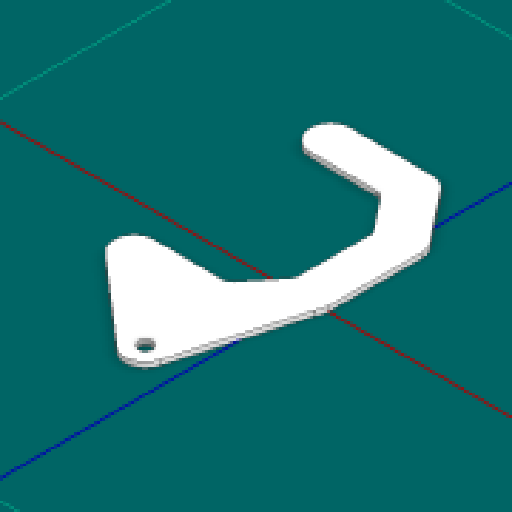
# Autodesk Inventor part: funnel_gusset
Saved by Autodesk Inventor 2025 (Build 290162000, 162)
## iProperties
Created: 2024-08-16
Part Number: funnel_gusset
Material: Acetal Resin, White
Document SubType Name: Modeling
Designer: averey
Density: 1.425 g/cm^3
Appearance: Smooth - White
d0: 0.500 in
d1: 0.500 in
d2: 0.500 in
d3: 0.125 in
d6: 0.176 in
d7: 0.176 in
d8: 0.176 in
d9: 0.176 in
d10: 0.500 in
d11: 0.500 in
d12: 0.250 in
d13: 0.250 in
d14: 0.625 in
d15: 0.625 in
d16: 0.500 in
Author: averey
Autodesk Inventor part; units mm, degrees
ref_plane "YZ Plane" through (0, 0, 0) normal (1, 0, 0) x (0, 1, 0)
ref_plane "XZ Plane" through (0, 0, 0) normal (0, 1, 0) x (-1, 0, 0)
ref_plane "XY Plane" through (0, 0, 0) normal (0, 0, 1) x (1, 0, 0)
sketch "main_gusset" plane through (0, 0, 0) normal (0, 0, 1) x (1, 0, 0)
  circle A0 centre (-10.4381, -28.24) radius 2.1844
  arc A1 (-15.3966, -32.2068) -> (-10.4381, -34.59) centre (-10.4381, -28.24) ccw
  circle A2 centre (-23.1381, -12.365) radius 2.0955
  line L0 (-16.7881, 12.8688) -> (-16.7881, -9.0238)
  line L1 (-29.4881, 16.21) -> (-29.4881, -12.365)
  arc A3 (-16.7881, -9.0238) -> (-16.0924, -11.0072) centre (-13.6131, -9.0238) ccw
  arc A4 (-29.4881, -12.365) -> (-28.0966, -16.3318) centre (-23.1381, -12.365) ccw
  line L2 (-16.0924, -11.0072) -> (-8.3394, -20.6984)
  arc A5 (-8.3394, -20.6984) -> (-5.8602, -21.89) centre (-5.8602, -18.715) ccw
  line L3 (-28.0966, -16.3318) -> (-15.3966, -32.2068)
  line L4 (-10.4381, -34.59) -> (14.9619, -34.59)
  circle A6 centre (-10.4381, 32.085) radius 2.1844
  circle A7 centre (14.9619, 32.0717) radius 2.1844
  arc A8 (-10.4381, 38.435) -> (-15.3966, 36.0518) centre (-10.4381, 32.085) ccw
  arc A9 (14.3804, 25.735) -> (14.9619, 38.435) centre (14.9619, 32.0717) ccw
  line L5 (14.9619, 38.435) -> (-10.4381, 38.435)
  circle A10 centre (-23.1381, 16.21) radius 2.0955
  line L6 (14.9619, 25.735) -> (-5.8602, 25.735)
  arc A11 (-16.0924, 14.8522) -> (-16.7881, 12.8688) centre (-13.6131, 12.8688) ccw
  arc A12 (-28.0966, 20.1768) -> (-29.4881, 16.21) centre (-23.1381, 16.21) ccw
  line L7 (-8.3394, 24.5434) -> (-16.0924, 14.8522)
  arc A13 (-5.8602, 25.735) -> (-8.3394, 24.5434) centre (-5.8602, 22.56) ccw
  line L8 (-28.0966, 20.1768) -> (-15.3966, 36.0518)
  circle A14 centre (14.9619, -28.24) radius 2.1844
  arc A15 (14.9619, -34.59) -> (14.9619, -21.89) centre (14.9619, -28.24) ccw
  line L9 (-5.8602, -21.89) -> (14.9619, -21.89)
  line L10 (0.0267, 34.3202) -> (4.4971, 34.3202)
  line L11 (4.4971, 34.3202) -> (4.4971, 29.8498)
  line L12 (4.4971, 29.8498) -> (0.0267, 29.8498)
  line L13 (0.0267, 29.8498) -> (0.0267, 34.3202)
  line L14 (0.0267, 34.3202) -> (4.4971, 29.8498) construction
  line L15 (4.4971, 34.3202) -> (0.0267, 29.8498) construction
  line L16 (0.0267, -26.0048) -> (4.4971, -26.0048)
  line L17 (4.4971, -26.0048) -> (4.4971, -30.4752)
  line L18 (4.4971, -30.4752) -> (0.0267, -30.4752)
  line L19 (0.0267, -30.4752) -> (0.0267, -26.0048)
  line L20 (0.0267, -26.0048) -> (4.4971, -30.4752) construction
  line L21 (4.4971, -26.0048) -> (0.0267, -30.4752) construction
  point P0 (-1.5323, 2.5213)
  point P1 (2.2619, 32.085)
  point P2 (2.2619, -28.24)
  dimension "d0" = 12.7
  dimension "d1" = 12.7
  dimension "d2" = 12.7
  dimension "d3" = 3.175
  dimension "d6" = 4.4704
  dimension "d7" = 4.4704
  dimension "d8" = 4.4704
  dimension "d9" = 4.4704
  dimension "d10" = 12.7
  dimension "d11" = 12.7
  dimension "d12" = 6.35
  dimension "d13" = 6.35
  dimension "d14" = 15.875
  dimension "d15" = 15.875
  dimension "d16" = 12.7
  measures "d0" diameter of A12
  measures "d1" diameter of A4
  measures "d2" distance between parallel lines of L8 L7
  measures "d3" radius of A11
  measures "d6" distance of L11.end L12.end
  measures "d7" distance of L10.end L11.end
  measures "d8" distance of L17.end L18.end
  measures "d9" distance of L16.end L17.end
  measures "d10" horizontal distance of A10.centre A6.centre
  measures "d11" horizontal distance of A2.centre A0.centre
  measures "d12" radius of A1
  measures "d13" radius of A8
  measures "d14" vertical distance of A2.centre A0.centre
  measures "d15" vertical distance of A6.centre A10.centre
  measures "d16" distance of A7.centre point (2.262, 32.085)
sketch "Sketch1" plane through (0, 0, 0) normal (0, 1, 0) x (-1, 0, 0)
  arc A0 (15.5751, 43.7797) -> (5.2982, 40.7397) centre (11.4031, 38.9925) ccw
  line L0 (42.3791, 20.4205) -> (15.5751, 43.7797)
  line L1 (-6.3499, 0.0397) -> (5.2982, 40.7397)
  circle A1 centre (11.4031, 38.9925) radius 2.1844 projected
  arc A2 (15.5751, 43.7797) -> (5.2982, 40.7397) centre (11.4031, 38.9925) ccw
  circle A3 centre (12.422, -44.5285) radius 2.1844
  arc A4 (7.4388, -48.4642) -> (12.3823, -50.8784) centre (12.422, -44.5285) ccw
  circle A5 centre (-0.1786, -28.5744) radius 2.0955
  line L2 (6.329, -3.3808) -> (6.1922, -25.273)
  line L3 (-6.3499, 0.0397) -> (-6.5284, -28.5348)
  arc A6 (6.1922, -25.273) -> (6.8755, -27.2607) centre (9.3671, -25.2928) ccw
  arc A7 (-6.5284, -28.5348) -> (-5.1618, -32.5102) centre (-0.1786, -28.5744) ccw
  line L4 (6.8755, -27.2607) -> (14.5678, -37.0002)
  arc A8 (14.5678, -37.0002) -> (17.0395, -38.2072) centre (17.0594, -35.0323) ccw
  line L5 (-5.1618, -32.5102) -> (7.4388, -48.4642)
  line L6 (12.3823, -50.8784) -> (37.7818, -51.0371)
  circle A9 centre (12.799, 15.7953) radius 2.1844
  circle A10 centre (38.1984, 15.6233) radius 2.1844
  arc A11 (12.8386, 22.1452) -> (7.8653, 19.793) centre (12.799, 15.7953) ccw
  arc A12 (37.5773, 9.2904) -> (38.2381, 21.9865) centre (38.1984, 15.6233) ccw
  line L7 (38.2381, 21.9865) -> (12.8386, 22.1452)
  circle A13 centre (0, 0) radius 2.0955
  line L8 (38.1588, 9.2867) -> (17.3371, 9.4168)
  arc A14 (7.0371, -1.4018) -> (6.329, -3.3808) centre (9.5039, -3.4006) ccw
  arc A15 (-4.9336, 3.9977) -> (-6.3499, 0.0397) centre (0, 0) ccw
  line L9 (14.8505, 8.2408) -> (7.0371, -1.4018)
  arc A16 (17.3371, 9.4168) -> (14.8505, 8.2408) centre (17.3173, 6.2419) ccw
  line L10 (-4.9336, 3.9977) -> (7.8653, 19.793)
  circle A17 centre (37.8215, -44.6872) radius 2.1844
  arc A18 (37.7818, -51.0371) -> (37.8612, -38.3374) centre (37.8215, -44.6872) ccw
  line L11 (17.0395, -38.2072) -> (37.8612, -38.3374)
  line L12 (23.2775, 17.9651) -> (27.7478, 17.9371)
  line L13 (27.7478, 17.9371) -> (27.7199, 13.4668)
  line L14 (27.7199, 13.4668) -> (23.2496, 13.4948)
  line L15 (23.2496, 13.4948) -> (23.2775, 17.9651)
  line L16 (23.2775, 17.9651) -> (27.7199, 13.4668) construction
  line L17 (27.7478, 17.9371) -> (23.2496, 13.4948) construction
  line L18 (22.9005, -42.3587) -> (27.3708, -42.3867)
  line L19 (27.3708, -42.3867) -> (27.3429, -46.857)
  line L20 (27.3429, -46.857) -> (22.8726, -46.8291)
  line L21 (22.8726, -46.8291) -> (22.9005, -42.3587)
  line L22 (22.9005, -42.3587) -> (27.3429, -46.857) construction
  line L23 (27.3708, -42.3867) -> (22.8726, -46.8291) construction
  point P0 (0, 0)
  point P1 (42.3791, 20.4205)
  point P2 (-6.3499, 0.0397)
  point P3 (-5.4094, 3.3258)
  point P4 (-6.3499, 0.0397)
  dimension "d18" = 12.7
  constraints: 4 end point, 4 point on circle, 3 tangent, 2 centre point, 2 coincident, 4 other
  measures "d18" diameter of A0
extrude "Extrusion1" add sketch "Sketch1" along normal blind 1.5875
body "Solid1"
